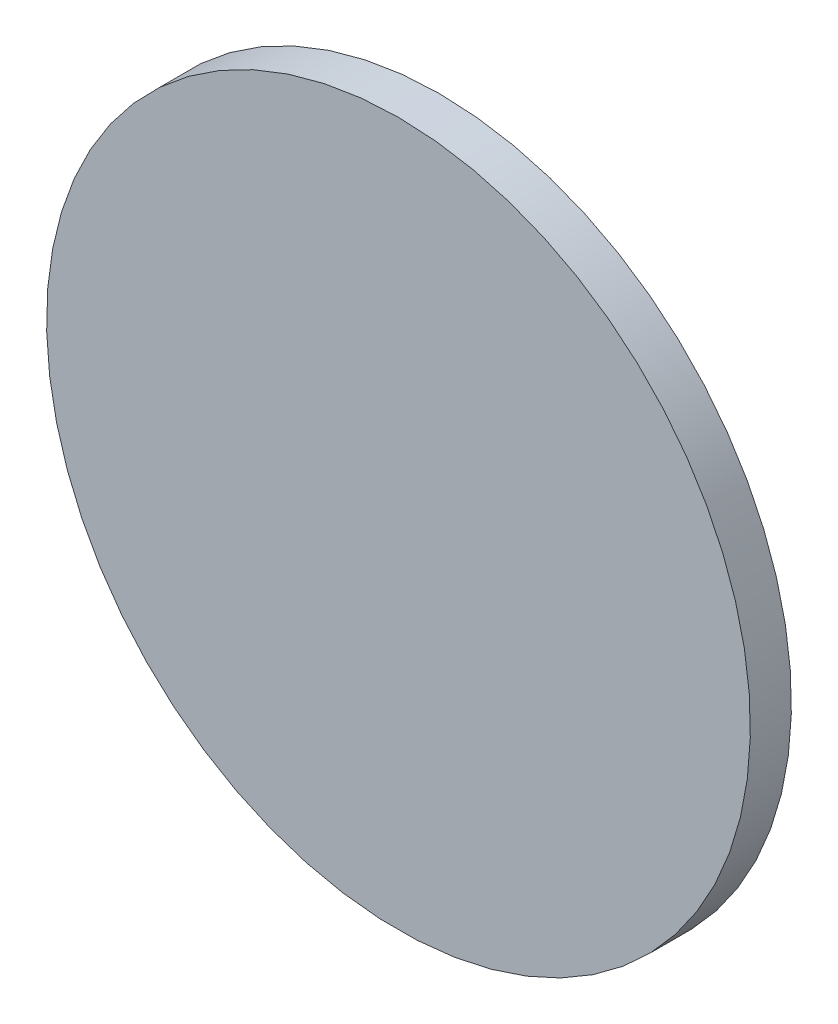
# Autodesk Inventor part: 50_ETL_Membrane_Mould_Lower_v0
Saved by Autodesk Inventor 2022 (Build 260153000, 153)
## iProperties
Created: 2021-12-31
Part Number: 50_ETL_Membrane_Mould_Lower_v0
Material: Generisch
Document SubType Name: Modeling
Designer: diederichbenedict
Density: 1 g/cm^3
Appearance: Türkis
Author: diederichbenedict
Autodesk Inventor part; units mm, degrees
ref_plane "YZ Plane" through (0, 0, 0) normal (1, 0, 0) x (0, 1, 0)
ref_plane "XZ Plane" through (0, 0, 0) normal (0, 1, 0) x (-1, 0, 0)
ref_plane "XY Plane" through (0, 0, 0) normal (0, 0, 1) x (1, 0, 0)
sketch "Skizze1" plane through (0, 0, 0) normal (1, 0, 0) x (0, 1, 0)
  line L0 (-20.6011, -1.9989) -> (-21.4, -1.2)
  line L1 (-21.4, -1.2) -> (-21.4, 0)
  line L2 (-25, 0) -> (-25, -0.6)
  line L3 (-22.8485, -0.6) -> (-20.8497, -2.5989)
  line L4 (0.345, -0.6) -> (5, -0.6)
  line L5 (5, -0.6) -> (5, 1.4)
  line L6 (-12.5, -6.6891) -> (-12.5, -2.8)
  line L7 (5, 1.4) -> (-12.155, 1.4)
  line L8 (-6.155, -0.8) -> (-6.155, -1) construction
  line L9 (-6.155, -1) -> (-18.155, -1) construction
  line L10 (-18.155, -1) -> (-18.155, -0.8) construction
  line L11 (-18.155, -0.8) -> (-13.2371, -0.918) construction
  line L12 (-12.155, 1.4) -> (-12.155, -0.7885)
  line L13 (-5.1181, -0.7885) -> (-5.1181, -1) construction
  line L14 (-5.1181, -0.7885) -> (-5.1181, -1) construction
  line L15 (-5.1181, -0.7885) -> (-5.1181, -1)
  line L16 (-6.155, -1) -> (-6.5167, -1)
  line L17 (-5.7914, -1.4086) -> (-6.1109, -1.0891)
  line L18 (-3.6, 0) -> (0, 0)
  line L19 (-5.7914, -1.4086) -> (-6.1109, -1.0891)
  line L20 (-19.1918, -1) -> (-5.1181, -1) projected
  line L21 (-5.1181, -0.7885) -> (-12.155, -0.7885)
  line L22 (-5.1181, -1) -> (-3.9212, -2.2)
  line L23 (-3.6692, -2.2) -> (-2.6692, -1.2) construction
  line L24 (-3.9212, -2.2) -> (-3.6692, -2.2)
  line L25 (-3.6692, -2.2) -> (-2.6692, -1.2)
  line L26 (-2.6692, -1.2) -> (-2.6692, 0)
  line L27 (0.345, 0) -> (0.345, -0.6) construction
  line L28 (0.345, -0.6) -> (0.345, 0)
  line L29 (0.345, 0) -> (-2.6692, 0)
  point P0 (0, -0.6)
  point P1 (-2.1515, -0.6)
  point P2 (-20.8023, -2.2)
  point P3 (-22.8485, -0.6)
  point P4 (-21.0508, -2.8)
  point P5 (-12.155, -1)
  point P6 (-5, -2.2)
  point P7 (-3.2, 0)
  dimension "d1" = 2
  constraints: 58 end point, 4 perpendicular, 4 vertical, 3 horizontal, 3 point on line, 1 collinear, 1 midpoint, 1 parallel, 18 other
  measures "d1" distance of L4.end L5.end
revolve "Umdrehung1" add sketch "Skizze1" angle 360 about axis through (0, -12.155, 1.4) along (0, 0, -1)
